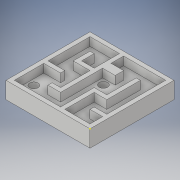
# Autodesk Inventor part: Part1
Saved by Autodesk Inventor 2018 (Build 220112000, 112)
## iProperties
Created: 2018-01-14
Part Number: Part1
Material: Generic
Document SubType Name: Modeling
Designer: Marlena Rehder
Density: 1 g/cm^3
Appearance: Default
Author: Marlena Rehder
Autodesk Inventor part; units mm, degrees
ref_plane "YZ Plane" through (0, 0, 0) normal (1, 0, 0) x (0, 1, 0)
ref_plane "XZ Plane" through (0, 0, 0) normal (0, 1, 0) x (-1, 0, 0)
ref_plane "XY Plane" through (0, 0, 0) normal (0, 0, 1) x (1, 0, 0)
sketch "Sketch1" plane through (0, 0, 0) normal (0, 1, 0) x (-1, 0, 0)
  line L0 (0, 0) -> (1000, 0)
  line L1 (1000, 0) -> (1000, -1000)
  line L2 (1000, -1000) -> (0, -1000)
  line L3 (0, -1000) -> (0, 0)
  dimension "d0" = 1000
  dimension "d1" = 1000
  dimension "d2" = 1000
  constraints: 8 end point, 1 horizontal, 1 perpendicular, 1 vertical
  measures "d0" distance of L0.start L0.end
  measures "d1" distance of L0.end L1.end
  measures "d2" distance of L1.end L2.end
extrude "Extrusion1" add sketch "Sketch1" along normal blind 500
sketch "Sketch2" plane through (0, 500, 0) normal (0, 1, 0) x (1, 0, 0)
  point P0 (0, 0)
sketch "Sketch3" plane through (0, 500, 0) normal (0, 1, 0) x (1, 0, 0)
  point P0 (0, 0)
sketch "Sketch4" plane through (0, 500, 0) normal (0, 1, 0) x (1, 0, 0)
  line L0 (-1000, 0) -> (0, 0) projected
  line L1 (-50, 50) -> (-50, 200)
  line L2 (-50, 200) -> (-200, 200)
  line L3 (-200, 200) -> (-350, 200)
  line L4 (-350, 200) -> (-350, 50)
  line L5 (-350, 50) -> (-50, 50)
  dimension "d7" = 150
  dimension "d8" = 150
  dimension "d9" = 150
  dimension "d10" = 150
  dimension "d13" = 200
  dimension "d14" = 50
  constraints: 10 end point, 2 perpendicular, 1 parallel, 1 point on line
  measures "d7" distance of L1.start L1.end
  measures "d8" distance of L1.end L2.end
  measures "d9" distance of L2.end L3.end
  measures "d10" distance of L3.end L4.end
  measures "d13" distance between parallel lines of L2 L0
  measures "d14" distance from line of L0.end L1
extrude "Extrusion2" cut sketch "Sketch4" against normal blind 100
sketch "Sketch5" plane through (0, 500, 0) normal (0, 1, 0) x (1, 0, 0)
  line L0 (-350, 200) -> (-50, 200) projected
  line L1 (-350, 200) -> (-350, 400)
  line L2 (-350, 400) -> (-50, 400)
  line L3 (-50, 400) -> (-50, 250)
  line L4 (-50, 250) -> (-200, 250)
  line L5 (-200, 250) -> (-200, 200)
  point P0 (0, 0)
  dimension "d17" = 200
  dimension "d18" = 300
  dimension "d19" = 150
  dimension "d20" = 150
  constraints: 10 end point, 3 perpendicular, 1 midpoint, 1 vertical
  measures "d17" distance of L0.start L1.end
  measures "d18" distance of L1.end L2.end
  measures "d19" distance of L2.end L3.end
  measures "d20" distance of L3.end L4.end
extrude "Extrusion3" cut sketch "Sketch5" against normal blind 100
sketch "Sketch6" plane through (0, 500, 0) normal (0, 1, 0) x (1, 0, 0)
  line L0 (-50, 400) -> (-50, 250) projected
  line L1 (-50, 400) -> (-50, 900)
  line L2 (-50, 900) -> (-50, 950)
  line L3 (-50, 950) -> (-550, 950)
  line L4 (-550, 950) -> (-550, 800)
  line L5 (-550, 800) -> (-250, 800)
  line L6 (-250, 800) -> (-200, 800)
  line L7 (-200, 800) -> (-200, 400)
  line L8 (-350, 400) -> (-50, 400) projected
  line L9 (-200, 400) -> (-50, 400)
  point P0 (0, 0)
  dimension "d23" = 500
  dimension "d24" = 50
  dimension "d25" = 500
  dimension "d26" = 150
  dimension "d27" = 300
  dimension "d28" = 50
  constraints: 16 end point, 3 perpendicular, 3 vertical, 1 collinear, 1 point on line
  measures "d23" distance of L0.start L1.end
  measures "d24" distance of L1.end L2.end
  measures "d25" distance of L2.end L3.end
  measures "d26" distance of L3.end L4.end
  measures "d27" distance of L4.end L5.end
  measures "d28" distance of L5.end L6.end
extrude "Extrusion4" cut sketch "Sketch6" against normal blind 100
sketch "Sketch7" plane through (0, 500, 0) normal (0, 1, 0) x (1, 0, 0)
  line L0 (-250, 800) -> (-250, 500)
  line L1 (-250, 500) -> (-250, 450)
  line L2 (-250, 450) -> (-400, 450)
  line L3 (-400, 450) -> (-400, 50)
  line L4 (-400, 50) -> (-550, 50)
  line L5 (-550, 50) -> (-550, 200)
  line L6 (-550, 200) -> (-550, 400)
  line L7 (-550, 400) -> (-550, 600)
  line L8 (-550, 600) -> (-550, 700)
  line L9 (-550, 700) -> (-400, 700)
  line L10 (-400, 700) -> (-400, 800)
  line L11 (-400, 800) -> (-250, 800)
  point P0 (0, 0)
  point P1 (-200, 800)
  dimension "d32" = 50
  dimension "d33" = 300
  dimension "d34" = 50
  dimension "d35" = 150
  dimension "d36" = 400
  dimension "d37" = 150
  dimension "d38" = 150
  dimension "d39" = 200
  dimension "d40" = 200
  dimension "d41" = 100
  dimension "d42" = 150
  dimension "d43" = 250
  constraints: 24 end point, 6 point on line, 4 perpendicular, 1 parallel, 1 vertical
  measures "d32" distance of point (-200, 800) L0.start
  measures "d33" distance of L0.start L0.end
  measures "d34" distance of L0.end L1.end
  measures "d35" distance of L1.end L2.end
  measures "d36" distance of L2.end L3.end
  measures "d37" distance of L3.end L4.end
  measures "d38" distance of L4.end L5.end
  measures "d39" distance of L5.end L6.end
  measures "d40" distance of L6.end L7.end
  measures "d41" distance of L7.end L8.end
  measures "d42" distance of L8.end L9.end
  measures "d43" distance from line of point (0, 0) L0
extrude "Extrusion5" cut sketch "Sketch7" against normal blind 100
sketch "Sketch8" plane through (0, 500, 0) normal (0, 1, 0) x (1, 0, 0)
  point P0 (0, 0)
sketch "Sketch9" plane through (0, 500, 0) normal (0, 1, 0) x (1, 0, 0)
  point P0 (0, 0)
sketch "Sketch10" plane through (0, 500, 0) normal (0, 1, 0) x (1, 0, 0)
  line L0 (0, 0) -> (0, 1000) projected
  line L1 (-550, 50) -> (-550, 200)
  line L2 (-550, 50) -> (-550, 700) projected
  line L3 (-550, 200) -> (-650, 200)
  line L4 (-650, 200) -> (-850, 200)
  line L5 (-850, 200) -> (-900, 200)
  line L6 (-900, 200) -> (-950, 200)
  line L7 (-950, 200) -> (-950, 50)
  line L8 (-950, 50) -> (-550, 50)
  point P0 (-400, 50)
  dimension "d48" = 150
  dimension "d49" = 150
  dimension "d50" = 100
  dimension "d51" = 200
  dimension "d52" = 50
  dimension "d53" = 50
  constraints: 14 end point, 4 point on line, 2 perpendicular, 1 horizontal
  measures "d48" distance of point (-400, 50) L1.start
  measures "d49" distance of L1.start L1.end
  measures "d50" distance of L1.end L3.end
  measures "d51" distance of L3.end L4.end
  measures "d52" distance of L4.end L5.end
  measures "d53" distance of L5.end L6.end
extrude "Extrusion6" cut sketch "Sketch10" against normal blind 100
sketch "Sketch11" plane through (0, 500, 0) normal (0, 1, 0) x (1, 0, 0)
  line L0 (-700, 200) -> (-700, 250)
  line L1 (-700, 250) -> (-600, 250)
  line L2 (-600, 250) -> (-600, 400)
  line L3 (-600, 400) -> (-950, 400)
  line L4 (-950, 400) -> (-950, 200)
  line L5 (-950, 200) -> (-700, 200)
  point P0 (0, 0)
  dimension "d60" = 50
  dimension "d61" = 100
  dimension "d62" = 150
  dimension "d63" = 350
  constraints: 12 end point, 3 perpendicular, 2 parallel, 1 vertical
  measures "d60" distance of L0.start L0.end
  measures "d61" distance of L0.end L1.end
  measures "d62" distance of L1.end L2.end
  measures "d63" distance of L2.end L3.end
extrude "Extrusion7" cut sketch "Sketch11" against normal blind 100
sketch "Sketch12" plane through (0, 500, 0) normal (0, 1, 0) x (1, 0, 0)
  point P0 (0, 0)
sketch "Sketch13" plane through (0, 500, 0) normal (0, 1, 0) x (1, 0, 0)
  line L0 (0, 0) -> (0, 1000) projected
  line L1 (-600, 400) -> (-600, 550)
  line L2 (-600, 550) -> (-600, 600)
  line L3 (-950, 600) -> (-950, 450)
  line L4 (-950, 450) -> (-750, 450)
  line L5 (-750, 450) -> (-750, 400)
  line L6 (-750, 400) -> (-600, 400)
  line L7 (-950, 600) -> (-950, 950)
  line L8 (-950, 950) -> (-650, 950)
  line L9 (-650, 950) -> (-600, 950)
  line L10 (-600, 950) -> (-600, 650)
  line L11 (-600, 650) -> (-750, 650)
  line L12 (-750, 650) -> (-750, 700)
  line L13 (-750, 700) -> (-750, 800)
  line L14 (-750, 800) -> (-800, 800)
  line L15 (-800, 800) -> (-800, 600)
  line L16 (-600, 600) -> (-600, 400)
  line L17 (-800, 600) -> (-600, 600)
  dimension "d69" = 150
  dimension "d70" = 50
  dimension "d71" = 350
  dimension "d72" = 150
  dimension "d73" = 200
  dimension "d74" = 350
  dimension "d75" = 300
  dimension "d76" = 50
  dimension "d77" = 300
  dimension "d79" = 50
  dimension "d80" = 100
  dimension "d81" = 50
  dimension "d82" = 90
  dimension "d83" = 600
  dimension "d84" = 750
  constraints: 34 end point, 6 perpendicular, 4 parallel, 3 point on line, 1 horizontal, 1 vertical
  measures "d69" distance of L1.start L1.end
  measures "d70" distance of L1.end L2.end
  measures "d71" distance of L2.end L3.start
  measures "d72" distance of L3.start L3.end
  measures "d73" distance of L3.end L4.end
  measures "d74" distance of L3.start L7.end
  measures "d75" distance of L7.end L8.end
  measures "d76" distance of L8.end L9.end
  measures "d77" distance of L9.end L10.end
  measures "d79" distance of L11.end L12.end
  measures "d80" distance of L12.end L13.end
  measures "d81" distance of L13.end L14.end
  measures "d82" angle of L9 L5
  measures "d83" distance between parallel lines of L10 L0
  measures "d84" distance between parallel lines of L12 L0
extrude "Extrusion8" cut sketch "Sketch13" against normal blind 100
sketch "Sketch14" plane through (0, 400, 0) normal (0, 1, 0) x (1, 0, 0)
  circle A0 centre (-882.0732, 213.6869) radius 50
  point P0 (0, 0)
  dimension "d87" = 100
  dimension "d88" = 907.5875
  constraints: 1 centre point
  measures "d87" diameter of A0
  measures "d88" distance of point (0, 0) A0.centre
extrude "Extrusion9" cut sketch "Sketch14" against normal blind 500
sketch "Sketch15" plane through (0, 400, 0) normal (0, 1, 0) x (1, 0, 0)
  circle A0 centre (-473.0021, 632.6041) radius 50
  point P0 (0, 0)
  dimension "d91" = 100
  dimension "d92" = 789.8854
  constraints: 1 centre point
  measures "d91" diameter of A0
  measures "d92" distance of point (0, 0) A0.centre
extrude "Extrusion10" cut sketch "Sketch15" against normal blind 500
sketch "Sketch16" plane through (0, 0, 0) normal (0, -1, 0) x (1, 0, 0)
  line L0 (0, -1000) -> (0, 0) projected
  line L1 (0, 0) -> (0, -1000)
  line L2 (0, -1000) -> (-1000, -1000)
  line L3 (-1000, -1000) -> (-1000, 0) projected
  line L4 (-1000, -1000) -> (-1000, 0)
  line L5 (-1000, 0) -> (0, 0) projected
  line L6 (-1000, 0) -> (0, 0)
  constraints: 8 end point, 3 collinear, 1 perpendicular
extrude "Extrusion11" cut sketch "Sketch16" against normal blind 300
body "Solid1"
